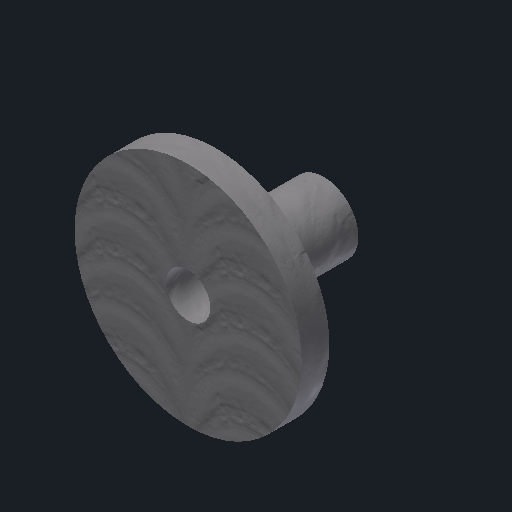
# Autodesk Inventor part: Tuerca3
Saved by Autodesk Inventor 2022 (Build 260153000, 153)
## iProperties
Created: 2021-09-20
Part Number: Tuerca3
Material: Steel, Mild, Welded
Document SubType Name: Modeling
Designer: Andres
Density: 7.85 g/cm^3
Appearance: Weld - Steel Mild
Author: Andres
Autodesk Inventor part; units mm, degrees
ref_plane "YZ Plane" through (0, 0, 0) normal (1, 0, 0) x (0, 1, 0)
ref_plane "XZ Plane" through (0, 0, 0) normal (0, 1, 0) x (-1, 0, 0)
ref_plane "XY Plane" through (0, 0, 0) normal (0, 0, 1) x (1, 0, 0)
sketch "Sketch1" plane through (0, 0, 0) normal (1, 0, 0) x (0, 1, 0)
  line L0 (0, -68.5665) -> (0, 42.4294) projected
  line L1 (0, 26.5728) -> (0, -52.7099)
  line L2 (-15, 2) -> (-15, -5)
  line L3 (-15, -5) -> (-12.5, -5)
  line L4 (-12.5, -5) -> (-12.5, -37)
  line L5 (-12.5, -37) -> (0, -37)
  line L6 (-15, 2) -> (-41, 2)
  line L7 (-41, 2) -> (-41, 12)
  line L8 (-41, 12) -> (0, 12)
  line L9 (-60, 0) -> (53.5817, 0) projected
  line L10 (-60, 10) -> (53.5817, 10) projected
  line L11 (-8, 12) -> (-8, -8)
  line L12 (-8, -8) -> (-10, -8)
  line L13 (-10, -8) -> (-10, -37)
  point P0 (0, 0)
  dimension "d1" = 82
  dimension "d2" = 2
  dimension "d3" = 10
  dimension "d4" = 25
  dimension "d5" = 30
  dimension "d8" = 20
  dimension "d11" = 16
  dimension "L_roscado" = 20
  dimension "d16" = 5
  dimension "d17" = 32
  constraints: 22 end point, 6 perpendicular, 6 point on line, 3 vertical, 1 horizontal
  measures "d1" diameter of L7 L1
  measures "d2" distance between parallel lines of L6 L9
  measures "d3" distance between parallel lines of L6 L8
  measures "d4" diameter of L4 L1
  measures "d5" diameter of L2 L1
  measures "d8" diameter of L13 L1
  measures "d11" diameter of L11 L1
  measures "L_roscado" distance between parallel lines of L8 L12
  measures "d16" distance between parallel lines of L9 L3
  measures "d17" distance between parallel lines of L3 L5
revolve "Revolution1" add sketch "Sketch1" angle 360 about axis through (0, 0, 26.5728) along (0, 0, -1) contours L5 L4 L3 L2 L9 L11 L12 L13 | L9 L2 L6 L7 L10 L11 | L10 L7 L8 L11
body "Solid1"
